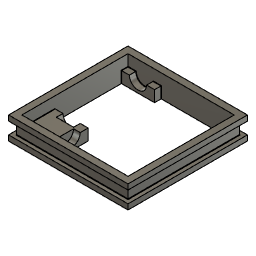
MTQ+support (Autodesk Fusion 360 design; units mm, degrees)
Autodesk Fusion 360 part; units mm, degrees
sketch "Sketch2" plane through (0, 0, 0) normal (0, 1, 0) x (1, 0, 0)
  line L0 (-45, 45) -> (45, 45)
  line L1 (45, 45) -> (45, -45)
  line L2 (45, -45) -> (-45, -45)
  line L3 (-45, -45) -> (-45, 45)
  line L4 (-45, 45) -> (45, -45) construction
  line L5 (45, 45) -> (-45, -45) construction
  line L6 (40, 40) -> (40, -40)
  line L7 (40, -40) -> (-40, -40)
  line L8 (-40, -40) -> (-40, 40)
  line L9 (-40, 40) -> (40, 40)
  line L10 (40, 0) -> (-40, 0) construction
  line L11 (-40, -40) -> (-15, -40)
  line L12 (-15, -40) -> (-15, -15)
  line L13 (-15, -15) -> (-40, -15)
  line L14 (-40, -15) -> (-40, -40)
  dimension "d1" = 90
  dimension "d2" = 90
  dimension "d109" = 80
  dimension "d110" = 80
  dimension "d111" = 25
  dimension "d112" = 25
  constraint horizontal L0
  constraint perpendicular L0 L1
  constraint parallel L0 L2
  constraint parallel L1 L3
  constraint coincident L4 origin
  constraint coincident L5 origin
  constraint vertical L6
  constraint coincident L1.end L2
  constraint vertical L8
  constraint equal L6 L8
  constraint horizontal L7
  constraint midpoint L6 L10.start
  constraint midpoint L8 L10.end
  constraint midpoint L5 L10
  constraint horizontal L11
  constraint vertical L12
  constraint horizontal L13
  constraint vertical L14
  measures "d1" distance of L1.end L2.end
  measures "d2" distance of L0.end L1.end
  measures "d109" distance of L6.end L7.end
  measures "d110" distance of L7.end L8.end
  measures "d111" distance of L7.end L11.end
  measures "d112" distance of L7.end L13.end
extrude "Extrude3" add sketch "Sketch2" along normal blind 17
sketch "Sketch7" plane through (0, 0, 0) normal (1, 0, 0) x (0, 0, -1)
  line L0 (42, 13) -> (45, 13)
  line L1 (45, 4) -> (42, 4)
  line L2 (42, 4) -> (42, 13)
  line L3 (45, 13) -> (45, 4)
  line L4 (45, 0) -> (45, 17)
  dimension "d79" = 3
  dimension "d80" = 9
  constraint horizontal L0
  constraint horizontal L1
  constraint vertical L2
  constraint perpendicular L1 L3
  constraint coincident L3 L4.start
  measures "d79" distance of L0.start L0.end
  measures "d80" distance of L0.start L1.end
sweep "Sweep2" cut profiles "Sketch7" along 4 edges at (0, 17, -45) (-45, 17, 0) (0, 17, 45) (45, 17, 0) section 1
sketch "Sketch9" plane through (0, 0, -40) normal (0, 0, 1) x (1, 0, 0)
  line L0 (-40, 0) -> (40, 0)
  line L1 (40, 0) -> (40, 17)
  line L2 (40, 17) -> (-40, 17)
  line L3 (-40, 17) -> (-40, 0)
  line L4 (-15, 8.5) -> (-15, 0)
  line L5 (-15, 0) -> (-40, 0)
  line L6 (-40, 0) -> (-40, 8.5)
  line L7 (-40, 17) -> (-15, 0) construction
  arc A0 (-34, 8.5) -> (-21, 8.5) centre (-27.5, 8.5) ccw
  line L8 (-40, 8.5) -> (-34, 8.5)
  line L9 (-21, 8.5) -> (-15, 8.5)
  line L10 (-34, 8.5) -> (-21, 8.5)
  line L11 (-40, 0) -> (-40, 17)
  dimension "d92" = 13
  dimension "d93" = 25
  dimension "d113" = 8.5
  constraint vertical L4
  constraint horizontal L5
  constraint vertical L6
  constraint coincident L0 L4.end
  constraint coincident L2.end L3.start
  constraint midpoint A0.centre L7
  constraint coincident A0.end L8
  constraint collinear L8 L9
  constraint collinear L3 L6
  measures "d92" diameter of A0
  measures "d93" distance of L4.end L0.start
  measures "d113" distance of L4.end L4.start
extrude "Extrude6" add sketch "Sketch9" along normal blind 5 contours L0 L3 L4 L5 L6 A0 L8 L9 L11
sketch "Sketch10" plane through (40, 0, 0) normal (-1, 0, 0) x (0, 0, 1)
  line L0 (-40, 0) -> (40, 0)
  line L1 (40, 17) -> (-40, 17)
  line L2 (-40, 17) -> (-40, 0)
  line L3 (15, 0) -> (15, 8.5)
  line L4 (40, 0) -> (15, 0)
  line L5 (40, 8.5) -> (40, 0)
  line L6 (-40, 17) -> (40, 17)
  line L7 (40, 0) -> (40, 17)
  line L8 (40, 8.5) -> (15, 8.5)
  arc A0 (21, 8.5) -> (34, 8.5) centre (27.5, 8.5) ccw
  dimension "d96" = 13
  dimension "d97" = 25
  dimension "d102" = 8.5
  constraint horizontal L4
  constraint vertical L3
  constraint coincident L0.end L4.start
  constraint coincident L5.start L7
  constraint coincident L5 L8.start
  constraint perpendicular L3 L8
  constraint midpoint A0.centre L8
  constraint coincident L8 A0.end
  constraint coincident L8 A0.start
  measures "d96" diameter of A0
  measures "d97" distance of L0.end L3.start
  measures "d102" distance of L3.end L3.start
extrude "Extrude7" add sketch "Sketch10" along normal blind 5 contours L0 L3 L4 L5 L7 L8 A0
extrude "Extrude8" add sketch "Sketch2" along normal blind 8.5 contours L7 L8 L11 L12 L13 L14
extrude "Extrude9" cut sketch "Sketch9" along normal blind 60 contours A0 L10
extrude "Extrude10" cut sketch "Sketch10" along normal blind 60 contours L8 A0
fillet "Fillet2" radius 0.25 8 edges at (42, 13, 0) (0, 13, -42) (-42, 13, 0) (0, 13, 42) (0, 4, -42) (42, 4, 0) (0, 4, 42) (-42, 4, 0)
fillet "Fillet3" radius 0.2 2 edges at (-40, 8.5, -37.5) (-37, 8.5, -40)
fillet "Fillet3" radius 0.2 12 edges at (-18, 8.5, -40) (-40, 8.5, 27.5) (-27.5, 8.5, 40) (37.5, 8.5, 40) (40, 8.5, 18) (40, 8.5, 37) (40, 4.25, 15) (35, 4.25, 40) (-15, 4.25, 40) (-40, 4.25, 15) (-40, 4.25, -35) (-15, 4.25, -40)
fillet "Fillet3" radius 0.2 2 edges at (-27.5, 2, -40) (40, 2, 27.5)
